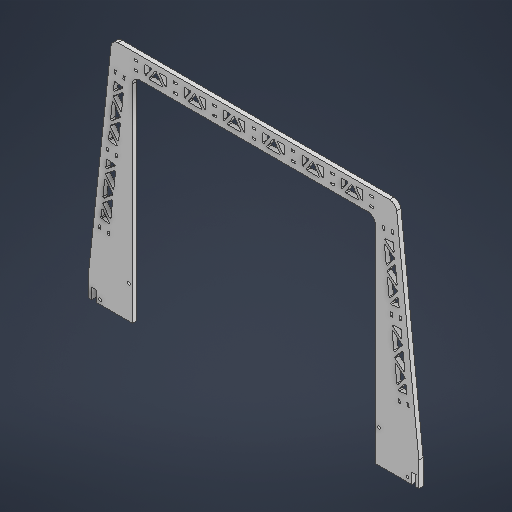
# Autodesk Inventor part: GateBrigeSideLessMaterial
Saved by Autodesk Inventor 2026 (Build 300175000, 175)
## iProperties
Created: 2025-03-30
Part Number: GateBrigeSideLessMaterial
Material: Všeobecné
Document SubType Name: Modeling
Designer: 42060
Density: 1 g/cm^3
Appearance: Výchozí
Author: 42060
Autodesk Inventor part; units mm, degrees
ref_plane "YZ Plane" through (0, 0, 0) normal (1, 0, 0) x (0, 1, 0)
ref_plane "XZ Plane" through (0, 0, 0) normal (0, 1, 0) x (-1, 0, 0)
ref_plane "XY Plane" through (0, 0, 0) normal (0, 0, 1) x (1, 0, 0)
sketch "Náčrt1" plane through (0, 0, 0) normal (0, 0, 1) x (1, 0, 0)
  line L0 (0, 0) -> (-160, 0)
  line L1 (-170, -10) -> (-170, -300)
  line L2 (-231, -300) -> (-231, -265.3)
  line L3 (-190.0581, 30) -> (0, 30)
  line L4 (0, 30) -> (0, 0)
  line L5 (-203.7, -249) -> (-170, -249)
  line L6 (-170, -249) -> (-170, -299)
  line L7 (-170, -299) -> (-220, -299)
  line L8 (-220, -299) -> (-220, -265.3)
  line L9 (-220, -265.3) -> (-203.7, -249)
  line L10 (-220, -299) -> (-170, -249) construction
  circle A0 centre (-215, -294) radius 2.1
  circle A1 centre (-175, -254) radius 2.1
  arc A2 (-160, 0) -> (-170, -10) centre (-160, -10) ccw
  line L11 (-200, 21.0762) -> (-231, -265.3)
  arc A3 (-190.0581, 30) -> (-200, 21.0762) centre (-190.0581, 20) ccw
  line L12 (-227, -300) -> (-227, -285)
  line L13 (-227, -285) -> (-221, -285)
  line L14 (-221, -285) -> (-221, -300)
  line L15 (-170, -300) -> (-221, -300)
  line L16 (-227, -300) -> (-231, -300)
  line L17 (0, 0) -> (160, 0)
  line L18 (170, -10) -> (170, -300)
  line L19 (231, -300) -> (231, -265.3)
  line L20 (190.0581, 30) -> (0, 30)
  line L21 (203.7, -249) -> (170, -249)
  line L22 (170, -249) -> (170, -299)
  line L23 (170, -299) -> (220, -299)
  line L24 (220, -299) -> (220, -265.3)
  line L25 (220, -265.3) -> (203.7, -249)
  line L26 (220, -299) -> (170, -249) construction
  circle A4 centre (215, -294) radius 2.1
  circle A5 centre (175, -254) radius 2.1
  arc A6 (170, -10) -> (160, 0) centre (160, -10) ccw
  line L27 (200, 21.0762) -> (231, -265.3)
  arc A7 (200, 21.0762) -> (190.0581, 30) centre (190.0581, 20) ccw
  line L28 (227, -300) -> (227, -285)
  line L29 (227, -285) -> (221, -285)
  line L30 (221, -285) -> (221, -300)
  line L31 (170, -300) -> (221, -300)
  line L32 (227, -300) -> (231, -300)
  line L33 (-36.6095, 9.0611) -> (-28.3278, 21.2788)
  line L34 (-26.6722, 21.2788) -> (-18.3905, 9.0611)
  line L35 (-19.2183, 7.5) -> (-35.7817, 7.5)
  line L36 (-21.6095, 20.9389) -> (-14.3278, 10.1964)
  line L37 (-12.5, 10.7575) -> (-12.5, 21.5)
  line L38 (-13.5, 22.5) -> (-20.7817, 22.5)
  line L39 (-33.3905, 20.9389) -> (-40.6722, 10.1964)
  line L40 (-42.5, 10.7575) -> (-42.5, 21.5)
  line L41 (-41.5, 22.5) -> (-34.2183, 22.5)
  line L42 (-55, 15) -> (0, 15) construction
  arc A8 (-41.5, 22.5) -> (-42.5, 21.5) centre (-41.5, 21.5) ccw
  arc A9 (-33.3905, 20.9389) -> (-34.2183, 22.5) centre (-34.2183, 21.5) ccw
  arc A10 (-42.5, 10.7575) -> (-40.6722, 10.1964) centre (-41.5, 10.7575) ccw
  arc A11 (-36.6095, 9.0611) -> (-35.7817, 7.5) centre (-35.7817, 8.5) ccw
  arc A12 (-19.2183, 7.5) -> (-18.3905, 9.0611) centre (-19.2183, 8.5) ccw
  arc A13 (-26.6722, 21.2788) -> (-28.3278, 21.2788) centre (-27.5, 20.7178) ccw
  arc A14 (-20.7817, 22.5) -> (-21.6095, 20.9389) centre (-20.7817, 21.5) ccw
  arc A15 (-12.5, 21.5) -> (-13.5, 22.5) centre (-13.5, 21.5) ccw
  arc A16 (-14.3278, 10.1964) -> (-12.5, 10.7575) centre (-13.5, 10.7575) ccw
  arc A17 (-81.6722, 21.2788) -> (-83.3278, 21.2788) centre (-82.5, 20.7178) ccw
  line L43 (-91.6095, 9.0611) -> (-83.3278, 21.2788)
  line L44 (-68.5, 22.5) -> (-75.7817, 22.5)
  arc A18 (-67.5, 21.5) -> (-68.5, 22.5) centre (-68.5, 21.5) ccw
  line L45 (-81.6722, 21.2788) -> (-73.3905, 9.0611)
  arc A19 (-74.2183, 7.5) -> (-73.3905, 9.0611) centre (-74.2183, 8.5) ccw
  line L46 (-76.6095, 20.9389) -> (-69.3278, 10.1964)
  line L47 (-74.2183, 7.5) -> (-90.7817, 7.5)
  arc A20 (-69.3278, 10.1964) -> (-67.5, 10.7575) centre (-68.5, 10.7575) ccw
  line L48 (-110, 15) -> (-55, 15) construction
  arc A21 (-96.5, 22.5) -> (-97.5, 21.5) centre (-96.5, 21.5) ccw
  arc A22 (-97.5, 10.7575) -> (-95.6722, 10.1964) centre (-96.5, 10.7575) ccw
  arc A23 (-91.6095, 9.0611) -> (-90.7817, 7.5) centre (-90.7817, 8.5) ccw
  arc A24 (-88.3905, 20.9389) -> (-89.2183, 22.5) centre (-89.2183, 21.5) ccw
  line L49 (-67.5, 10.7575) -> (-67.5, 21.5)
  arc A25 (-75.7817, 22.5) -> (-76.6095, 20.9389) centre (-75.7817, 21.5) ccw
  line L50 (-96.5, 22.5) -> (-89.2183, 22.5)
  line L51 (-88.3905, 20.9389) -> (-95.6722, 10.1964)
  line L52 (-97.5, 10.7575) -> (-97.5, 21.5)
  arc A26 (-136.6722, 21.2788) -> (-138.3278, 21.2788) centre (-137.5, 20.7178) ccw
  line L53 (-146.6095, 9.0611) -> (-138.3278, 21.2788)
  line L54 (-123.5, 22.5) -> (-130.7817, 22.5)
  arc A27 (-122.5, 21.5) -> (-123.5, 22.5) centre (-123.5, 21.5) ccw
  line L55 (-136.6722, 21.2788) -> (-128.3905, 9.0611)
  arc A28 (-129.2183, 7.5) -> (-128.3905, 9.0611) centre (-129.2183, 8.5) ccw
  line L56 (-131.6095, 20.9389) -> (-124.3278, 10.1964)
  line L57 (-129.2183, 7.5) -> (-145.7817, 7.5)
  arc A29 (-124.3278, 10.1964) -> (-122.5, 10.7575) centre (-123.5, 10.7575) ccw
  line L58 (-165, 15) -> (-110, 15) construction
  arc A30 (-151.5, 22.5) -> (-152.5, 21.5) centre (-151.5, 21.5) ccw
  arc A31 (-152.5, 10.7575) -> (-150.6722, 10.1964) centre (-151.5, 10.7575) ccw
  arc A32 (-146.6095, 9.0611) -> (-145.7817, 7.5) centre (-145.7817, 8.5) ccw
  arc A33 (-143.3905, 20.9389) -> (-144.2183, 22.5) centre (-144.2183, 21.5) ccw
  line L59 (-122.5, 10.7575) -> (-122.5, 21.5)
  arc A34 (-130.7817, 22.5) -> (-131.6095, 20.9389) centre (-130.7817, 21.5) ccw
  line L60 (-151.5, 22.5) -> (-144.2183, 22.5)
  line L61 (-143.3905, 20.9389) -> (-150.6722, 10.1964)
  line L62 (-152.5, 10.7575) -> (-152.5, 21.5)
  line L63 (-194.2882, -19.4076) -> (-184.4169, -20.4762)
  line L64 (-183.8976, -22.2495) -> (-194.8375, -31.0522)
  line L65 (-196.4586, -30.1655) -> (-195.39, -20.2942)
  line L66 (-182.8853, -28.7602) -> (-185.2377, -50.4911)
  line L67 (-187.011, -51.0104) -> (-196.7003, -38.9688)
  line L68 (-196.5481, -37.5628) -> (-184.5064, -27.8735)
  line L69 (-196.4225, -45.6946) -> (-186.7332, -57.7362)
  line L70 (-186.8854, -59.1422) -> (-198.927, -68.8315)
  line L71 (-200.5481, -67.9448) -> (-198.1958, -46.2139)
  line L72 (-188.596, -65.6528) -> (-200.6376, -75.3421)
  line L73 (-200.7898, -76.7481) -> (-191.1006, -88.7897)
  line L74 (-189.3273, -88.2704) -> (-186.9749, -66.5395)
  line L75 (-200.5121, -83.4739) -> (-191.7094, -94.4137)
  line L76 (-192.5961, -96.0348) -> (-202.4673, -94.9662)
  line L77 (-203.3539, -93.8644) -> (-202.2854, -83.9932)
  line L78 (-189.3526, -19.9419) -> (-188.3302, -10.4971) construction
  arc A35 (-194.2882, -19.4076) -> (-195.39, -20.2942) centre (-194.3958, -20.4018) ccw
  arc A36 (-183.8976, -22.2495) -> (-184.4169, -20.4762) centre (-184.5245, -21.4704) ccw
  arc A37 (-196.4586, -30.1655) -> (-194.8375, -31.0522) centre (-195.4644, -30.2731) ccw
  arc A38 (-196.5481, -37.5628) -> (-196.7003, -38.9688) centre (-195.9212, -38.3419) ccw
  arc A39 (-187.011, -51.0104) -> (-185.2377, -50.4911) centre (-186.2319, -50.3835) ccw
  arc A40 (-182.8853, -28.7602) -> (-184.5064, -27.8735) centre (-183.8795, -28.6526) ccw
  arc A41 (-196.4225, -45.6946) -> (-198.1958, -46.2139) centre (-197.2016, -46.3215) ccw
  arc A42 (-186.8854, -59.1422) -> (-186.7332, -57.7362) centre (-187.5123, -58.3631) ccw
  arc A43 (-200.5481, -67.9448) -> (-198.927, -68.8315) centre (-199.5539, -68.0524) ccw
  arc A44 (-200.6376, -75.3421) -> (-200.7898, -76.7481) centre (-200.0107, -76.1212) ccw
  arc A45 (-191.1006, -88.7897) -> (-189.3273, -88.2704) centre (-190.3215, -88.1628) ccw
  arc A46 (-186.9749, -66.5395) -> (-188.596, -65.6528) centre (-187.9691, -66.4319) ccw
  arc A47 (-200.5121, -83.4739) -> (-202.2854, -83.9932) centre (-201.2912, -84.1008) ccw
  arc A48 (-203.3539, -93.8644) -> (-202.4673, -94.9662) centre (-202.3597, -93.972) ccw
  arc A49 (-192.5961, -96.0348) -> (-191.7094, -94.4137) centre (-192.4885, -95.0406) ccw
  arc A50 (-214.116, -193.2836) -> (-213.2294, -194.3854) centre (-213.1218, -193.3913) ccw
  line L79 (-203.3581, -195.454) -> (-213.2294, -194.3854)
  arc A51 (-203.3581, -195.454) -> (-202.4714, -193.8329) centre (-203.2505, -194.4598) ccw
  arc A52 (-201.8626, -188.2089) -> (-200.0893, -187.6896) centre (-201.0835, -187.582) ccw
  line L80 (-211.2741, -182.8931) -> (-202.4714, -193.8329)
  line L81 (-214.116, -193.2836) -> (-213.0474, -183.4124)
  arc A53 (-211.2741, -182.8931) -> (-213.0474, -183.4124) centre (-212.0532, -183.52) ccw
  line L82 (-199.3581, -165.072) -> (-211.3997, -174.7613)
  line L83 (-211.5519, -176.1673) -> (-201.8626, -188.2089)
  line L84 (-200.0893, -187.6896) -> (-197.737, -165.9587)
  arc A54 (-211.3997, -174.7613) -> (-211.5519, -176.1673) centre (-210.7728, -175.5404) ccw
  arc A55 (-211.3102, -167.364) -> (-209.6891, -168.2507) centre (-210.316, -167.4716) ccw
  arc A56 (-197.737, -165.9587) -> (-199.3581, -165.072) centre (-198.7312, -165.8511) ccw
  line L85 (-207.1845, -145.1138) -> (-197.4953, -157.1554)
  arc A57 (-197.6475, -158.5614) -> (-197.4953, -157.1554) centre (-198.2744, -157.7823) ccw
  line L86 (-211.3102, -167.364) -> (-208.9578, -145.6331)
  line L87 (-197.6475, -158.5614) -> (-209.6891, -168.2507)
  arc A58 (-197.773, -150.4296) -> (-195.9997, -149.9103) centre (-196.9939, -149.8027) ccw
  arc A59 (-207.1845, -145.1138) -> (-208.9578, -145.6331) centre (-207.9636, -145.7407) ccw
  line L88 (-197.773, -150.4296) -> (-207.4623, -138.388)
  arc A60 (-207.3101, -136.982) -> (-207.4623, -138.388) centre (-206.6832, -137.7611) ccw
  arc A61 (-207.2206, -129.5847) -> (-205.5995, -130.4714) centre (-206.2264, -129.6923) ccw
  line L89 (-193.6474, -128.1794) -> (-195.9997, -149.9103)
  line L90 (-207.3101, -136.982) -> (-195.2685, -127.2927)
  arc A62 (-193.6474, -128.1794) -> (-195.2685, -127.2927) centre (-194.6416, -128.0718) ccw
  arc A63 (-194.6597, -121.6687) -> (-195.179, -119.8954) centre (-195.2866, -120.8896) ccw
  line L91 (-200.1146, -119.3611) -> (-199.0922, -109.9163) construction
  line L92 (-205.0502, -118.8268) -> (-195.179, -119.8954)
  arc A64 (-205.0502, -118.8268) -> (-206.152, -119.7134) centre (-205.1579, -119.821) ccw
  line L93 (-194.6597, -121.6687) -> (-205.5995, -130.4714)
  line L94 (-207.2206, -129.5847) -> (-206.152, -119.7134)
  line L95 (36.6095, 9.0611) -> (28.3278, 21.2788)
  line L96 (26.6722, 21.2788) -> (18.3905, 9.0611)
  line L97 (19.2183, 7.5) -> (35.7817, 7.5)
  line L98 (21.6095, 20.9389) -> (14.3278, 10.1964)
  line L99 (12.5, 10.7575) -> (12.5, 21.5)
  line L100 (13.5, 22.5) -> (20.7817, 22.5)
  line L101 (33.3905, 20.9389) -> (40.6722, 10.1964)
  line L102 (42.5, 10.7575) -> (42.5, 21.5)
  line L103 (41.5, 22.5) -> (34.2183, 22.5)
  line L104 (55, 15) -> (0, 15) construction
  arc A65 (42.5, 21.5) -> (41.5, 22.5) centre (41.5, 21.5) ccw
  arc A66 (34.2183, 22.5) -> (33.3905, 20.9389) centre (34.2183, 21.5) ccw
  arc A67 (40.6722, 10.1964) -> (42.5, 10.7575) centre (41.5, 10.7575) ccw
  arc A68 (35.7817, 7.5) -> (36.6095, 9.0611) centre (35.7817, 8.5) ccw
  arc A69 (18.3905, 9.0611) -> (19.2183, 7.5) centre (19.2183, 8.5) ccw
  arc A70 (28.3278, 21.2788) -> (26.6722, 21.2788) centre (27.5, 20.7178) ccw
  arc A71 (21.6095, 20.9389) -> (20.7817, 22.5) centre (20.7817, 21.5) ccw
  arc A72 (13.5, 22.5) -> (12.5, 21.5) centre (13.5, 21.5) ccw
  arc A73 (12.5, 10.7575) -> (14.3278, 10.1964) centre (13.5, 10.7575) ccw
  line L105 (67.5, 10.7575) -> (67.5, 21.5)
  line L106 (96.5, 22.5) -> (89.2183, 22.5)
  arc A74 (97.5, 21.5) -> (96.5, 22.5) centre (96.5, 21.5) ccw
  line L107 (97.5, 10.7575) -> (97.5, 21.5)
  arc A75 (95.6722, 10.1964) -> (97.5, 10.7575) centre (96.5, 10.7575) ccw
  arc A76 (67.5, 10.7575) -> (69.3278, 10.1964) centre (68.5, 10.7575) ccw
  arc A77 (68.5, 22.5) -> (67.5, 21.5) centre (68.5, 21.5) ccw
  arc A78 (89.2183, 22.5) -> (88.3905, 20.9389) centre (89.2183, 21.5) ccw
  arc A79 (83.3278, 21.2788) -> (81.6722, 21.2788) centre (82.5, 20.7178) ccw
  line L108 (88.3905, 20.9389) -> (95.6722, 10.1964)
  line L109 (91.6095, 9.0611) -> (83.3278, 21.2788)
  arc A80 (76.6095, 20.9389) -> (75.7817, 22.5) centre (75.7817, 21.5) ccw
  arc A81 (90.7817, 7.5) -> (91.6095, 9.0611) centre (90.7817, 8.5) ccw
  line L110 (110, 15) -> (55, 15) construction
  line L111 (68.5, 22.5) -> (75.7817, 22.5)
  line L112 (76.6095, 20.9389) -> (69.3278, 10.1964)
  line L113 (81.6722, 21.2788) -> (73.3905, 9.0611)
  arc A82 (73.3905, 9.0611) -> (74.2183, 7.5) centre (74.2183, 8.5) ccw
  line L114 (74.2183, 7.5) -> (90.7817, 7.5)
  line L115 (122.5, 10.7575) -> (122.5, 21.5)
  line L116 (151.5, 22.5) -> (144.2183, 22.5)
  arc A83 (152.5, 21.5) -> (151.5, 22.5) centre (151.5, 21.5) ccw
  line L117 (152.5, 10.7575) -> (152.5, 21.5)
  arc A84 (150.6722, 10.1964) -> (152.5, 10.7575) centre (151.5, 10.7575) ccw
  arc A85 (122.5, 10.7575) -> (124.3278, 10.1964) centre (123.5, 10.7575) ccw
  arc A86 (123.5, 22.5) -> (122.5, 21.5) centre (123.5, 21.5) ccw
  arc A87 (144.2183, 22.5) -> (143.3905, 20.9389) centre (144.2183, 21.5) ccw
  arc A88 (138.3278, 21.2788) -> (136.6722, 21.2788) centre (137.5, 20.7178) ccw
  line L118 (143.3905, 20.9389) -> (150.6722, 10.1964)
  line L119 (146.6095, 9.0611) -> (138.3278, 21.2788)
  arc A89 (131.6095, 20.9389) -> (130.7817, 22.5) centre (130.7817, 21.5) ccw
  arc A90 (145.7817, 7.5) -> (146.6095, 9.0611) centre (145.7817, 8.5) ccw
  line L120 (165, 15) -> (110, 15) construction
  line L121 (123.5, 22.5) -> (130.7817, 22.5)
  line L122 (131.6095, 20.9389) -> (124.3278, 10.1964)
  line L123 (136.6722, 21.2788) -> (128.3905, 9.0611)
  arc A91 (128.3905, 9.0611) -> (129.2183, 7.5) centre (129.2183, 8.5) ccw
  line L124 (129.2183, 7.5) -> (145.7817, 7.5)
  line L125 (194.2882, -19.4076) -> (184.4169, -20.4762)
  line L126 (183.8976, -22.2495) -> (194.8375, -31.0522)
  line L127 (196.4586, -30.1655) -> (195.39, -20.2942)
  line L128 (182.8853, -28.7602) -> (185.2377, -50.4911)
  line L129 (187.011, -51.0104) -> (196.7003, -38.9688)
  line L130 (196.5481, -37.5628) -> (184.5064, -27.8735)
  line L131 (196.4225, -45.6946) -> (186.7332, -57.7362)
  line L132 (186.8854, -59.1422) -> (198.927, -68.8315)
  line L133 (200.5481, -67.9448) -> (198.1958, -46.2139)
  line L134 (188.596, -65.6528) -> (200.6376, -75.3421)
  line L135 (200.7898, -76.7481) -> (191.1006, -88.7897)
  line L136 (189.3273, -88.2704) -> (186.9749, -66.5395)
  line L137 (200.5121, -83.4739) -> (191.7094, -94.4137)
  line L138 (192.5961, -96.0348) -> (202.4673, -94.9662)
  line L139 (203.3539, -93.8644) -> (202.2854, -83.9932)
  arc A92 (195.39, -20.2942) -> (194.2882, -19.4076) centre (194.3958, -20.4018) ccw
  arc A93 (184.4169, -20.4762) -> (183.8976, -22.2495) centre (184.5245, -21.4704) ccw
  arc A94 (194.8375, -31.0522) -> (196.4586, -30.1655) centre (195.4644, -30.2731) ccw
  arc A95 (196.7003, -38.9688) -> (196.5481, -37.5628) centre (195.9212, -38.3419) ccw
  arc A96 (185.2377, -50.4911) -> (187.011, -51.0104) centre (186.2319, -50.3835) ccw
  arc A97 (184.5064, -27.8735) -> (182.8853, -28.7602) centre (183.8795, -28.6526) ccw
  arc A98 (198.1958, -46.2139) -> (196.4225, -45.6946) centre (197.2016, -46.3215) ccw
  arc A99 (186.7332, -57.7362) -> (186.8854, -59.1422) centre (187.5123, -58.3631) ccw
  arc A100 (198.927, -68.8315) -> (200.5481, -67.9448) centre (199.5539, -68.0524) ccw
  arc A101 (200.7898, -76.7481) -> (200.6376, -75.3421) centre (200.0107, -76.1212) ccw
  arc A102 (189.3273, -88.2704) -> (191.1006, -88.7897) centre (190.3215, -88.1628) ccw
  arc A103 (188.596, -65.6528) -> (186.9749, -66.5395) centre (187.9691, -66.4319) ccw
  arc A104 (202.2854, -83.9932) -> (200.5121, -83.4739) centre (201.2912, -84.1008) ccw
  arc A105 (202.4673, -94.9662) -> (203.3539, -93.8644) centre (202.3597, -93.972) ccw
  arc A106 (191.7094, -94.4137) -> (192.5961, -96.0348) centre (192.4885, -95.0406) ccw
  arc A107 (195.179, -119.8954) -> (194.6597, -121.6687) centre (195.2866, -120.8896) ccw
  arc A108 (195.2685, -127.2927) -> (193.6474, -128.1794) centre (194.6416, -128.0718) ccw
  line L140 (205.0502, -118.8268) -> (195.179, -119.8954)
  line L141 (194.6597, -121.6687) -> (205.5995, -130.4714)
  line L142 (207.2206, -129.5847) -> (206.152, -119.7134)
  line L143 (207.3101, -136.982) -> (195.2685, -127.2927)
  arc A109 (206.152, -119.7134) -> (205.0502, -118.8268) centre (205.1579, -119.821) ccw
  arc A110 (205.5995, -130.4714) -> (207.2206, -129.5847) centre (206.2264, -129.6923) ccw
  line L144 (193.6474, -128.1794) -> (195.9997, -149.9103)
  arc A111 (208.9578, -145.6331) -> (207.1845, -145.1138) centre (207.9636, -145.7407) ccw
  line L145 (197.773, -150.4296) -> (207.4623, -138.388)
  arc A112 (207.4623, -138.388) -> (207.3101, -136.982) centre (206.6832, -137.7611) ccw
  arc A113 (195.9997, -149.9103) -> (197.773, -150.4296) centre (196.9939, -149.8027) ccw
  line L146 (207.1845, -145.1138) -> (197.4953, -157.1554)
  arc A114 (197.4953, -157.1554) -> (197.6475, -158.5614) centre (198.2744, -157.7823) ccw
  arc A115 (199.3581, -165.072) -> (197.737, -165.9587) centre (198.7312, -165.8511) ccw
  line L147 (197.6475, -158.5614) -> (209.6891, -168.2507)
  arc A116 (209.6891, -168.2507) -> (211.3102, -167.364) centre (210.316, -167.4716) ccw
  line L148 (211.3102, -167.364) -> (208.9578, -145.6331)
  arc A117 (202.4714, -193.8329) -> (203.3581, -195.454) centre (203.2505, -194.4598) ccw
  arc A118 (213.2294, -194.3854) -> (214.116, -193.2836) centre (213.1218, -193.3913) ccw
  arc A119 (200.0893, -187.6896) -> (201.8626, -188.2089) centre (201.0835, -187.582) ccw
  line L149 (214.116, -193.2836) -> (213.0474, -183.4124)
  line L150 (211.2741, -182.8931) -> (202.4714, -193.8329)
  arc A120 (213.0474, -183.4124) -> (211.2741, -182.8931) centre (212.0532, -183.52) ccw
  line L151 (211.5519, -176.1673) -> (201.8626, -188.2089)
  arc A121 (211.5519, -176.1673) -> (211.3997, -174.7613) centre (210.7728, -175.5404) ccw
  line L152 (200.0893, -187.6896) -> (197.737, -165.9587)
  line L153 (199.3581, -165.072) -> (211.3997, -174.7613)
  line L154 (203.3581, -195.454) -> (213.2294, -194.3854)
  line L155 (-2.5, 10) -> (2.5, 10)
  line L156 (2.5, 10) -> (2.5, 7.5)
  line L157 (2.5, 7.5) -> (-2.5, 7.5)
  line L158 (-2.5, 7.5) -> (-2.5, 10)
  line L159 (-2.5, 22.5) -> (2.5, 22.5)
  line L160 (2.5, 22.5) -> (2.5, 20)
  line L161 (2.5, 20) -> (-2.5, 20)
  line L162 (-2.5, 20) -> (-2.5, 22.5)
  line L163 (0, 20) -> (0, 10) construction
  line L164 (-42.5, 10.7575) -> (-42.5, 7.5) construction
  line L165 (-42.5, 7.5) -> (-40.6722, 10.1964) construction
  line L166 (-27.5, 22.5) -> (-27.5, 7.5) construction
  line L167 (-52.5, 10) -> (-52.5, 7.5)
  line L168 (-57.5, 10) -> (-52.5, 10)
  line L169 (-52.5, 7.5) -> (-57.5, 7.5)
  line L170 (-57.5, 7.5) -> (-57.5, 10)
  line L171 (-57.5, 22.5) -> (-52.5, 22.5)
  line L172 (-52.5, 20) -> (-57.5, 20)
  line L173 (-57.5, 20) -> (-57.5, 22.5)
  line L174 (-52.5, 22.5) -> (-52.5, 20)
  line L175 (-107.5, 10) -> (-107.5, 7.5)
  line L176 (-112.5, 10) -> (-107.5, 10)
  line L177 (-107.5, 7.5) -> (-112.5, 7.5)
  line L178 (-112.5, 7.5) -> (-112.5, 10)
  line L179 (-112.5, 22.5) -> (-107.5, 22.5)
  line L180 (-107.5, 20) -> (-112.5, 20)
  line L181 (-112.5, 20) -> (-112.5, 22.5)
  line L182 (-107.5, 22.5) -> (-107.5, 20)
  line L183 (-162.5, 10) -> (-162.5, 7.5)
  line L184 (-167.5, 10) -> (-162.5, 10)
  line L185 (-162.5, 7.5) -> (-167.5, 7.5)
  line L186 (-167.5, 7.5) -> (-167.5, 10)
  line L187 (-167.5, 22.5) -> (-162.5, 22.5)
  line L188 (-162.5, 20) -> (-167.5, 20)
  line L189 (-167.5, 20) -> (-167.5, 22.5)
  line L190 (-162.5, 22.5) -> (-162.5, 20)
  line L191 (52.5, 20) -> (52.5, 22.5)
  line L192 (57.5, 20) -> (52.5, 20)
  line L193 (57.5, 22.5) -> (57.5, 20)
  line L194 (52.5, 22.5) -> (57.5, 22.5)
  line L195 (57.5, 10) -> (57.5, 7.5)
  line L196 (52.5, 10) -> (57.5, 10)
  line L197 (57.5, 7.5) -> (52.5, 7.5)
  line L198 (52.5, 7.5) -> (52.5, 10)
  line L199 (107.5, 20) -> (107.5, 22.5)
  line L200 (112.5, 20) -> (107.5, 20)
  line L201 (112.5, 22.5) -> (112.5, 20)
  line L202 (107.5, 22.5) -> (112.5, 22.5)
  line L203 (112.5, 10) -> (112.5, 7.5)
  line L204 (107.5, 10) -> (112.5, 10)
  line L205 (112.5, 7.5) -> (107.5, 7.5)
  line L206 (107.5, 7.5) -> (107.5, 10)
  line L207 (162.5, 20) -> (162.5, 22.5)
  line L208 (167.5, 20) -> (162.5, 20)
  line L209 (167.5, 22.5) -> (167.5, 20)
  line L210 (162.5, 22.5) -> (167.5, 22.5)
  line L211 (167.5, 10) -> (167.5, 7.5)
  line L212 (162.5, 10) -> (167.5, 10)
  line L213 (167.5, 7.5) -> (162.5, 7.5)
  line L214 (162.5, 7.5) -> (162.5, 10)
  line L215 (-195.2485, -4.719) -> (-192.763, -4.988)
  line L216 (-192.763, -4.988) -> (-193.3011, -9.959)
  line L217 (-193.3011, -9.959) -> (-195.7866, -9.6899)
  line L218 (-195.7866, -9.6899) -> (-195.2485, -4.719)
  line L219 (-182.8211, -6.0642) -> (-180.3356, -6.3333)
  line L220 (-180.3356, -6.3333) -> (-180.8737, -11.3042)
  line L221 (-180.8737, -11.3042) -> (-183.3592, -11.0352)
  line L222 (-183.3592, -11.0352) -> (-182.8211, -6.0642)
  line L223 (-193.3011, -9.959) -> (-183.3592, -11.0352) construction
  line L224 (-206.5486, -109.1091) -> (-206.0105, -104.1382)
  line L225 (-203.5251, -104.4072) -> (-204.0632, -109.3782)
  line L226 (-204.0632, -109.3782) -> (-206.5486, -109.1091)
  line L227 (-206.0105, -104.1382) -> (-203.5251, -104.4072)
  line L228 (-194.1212, -110.4544) -> (-193.5831, -105.4834)
  line L229 (-191.6358, -110.7235) -> (-194.1212, -110.4544)
  line L230 (-191.0977, -105.7525) -> (-191.6358, -110.7235)
  line L231 (-193.5831, -105.4834) -> (-191.0977, -105.7525)
  line L232 (-204.0632, -109.3782) -> (-194.1212, -110.4544) construction
  line L233 (-203.5251, -104.4072) -> (-193.5831, -105.4834) construction
  line L234 (-198.6079, -105.4424) -> (-197.5317, -95.5005) construction
  line L235 (-217.3107, -208.5284) -> (-216.7726, -203.5574)
  line L236 (-214.2871, -203.8264) -> (-214.8252, -208.7974)
  line L237 (-214.8252, -208.7974) -> (-217.3107, -208.5284)
  line L238 (-216.7726, -203.5574) -> (-214.2871, -203.8264)
  line L239 (-204.8833, -209.8736) -> (-204.3452, -204.9026)
  line L240 (-202.3978, -210.1427) -> (-204.8833, -209.8736)
  line L241 (-201.8597, -205.1717) -> (-202.3978, -210.1427)
  line L242 (-204.3452, -204.9026) -> (-201.8597, -205.1717)
  line L243 (-214.8252, -208.7974) -> (-204.8833, -209.8736) construction
  line L244 (195.2485, -4.719) -> (192.763, -4.988)
  line L245 (192.763, -4.988) -> (193.3011, -9.959)
  line L246 (193.3011, -9.959) -> (195.7866, -9.6899)
  line L247 (195.7866, -9.6899) -> (195.2485, -4.719)
  line L248 (182.8211, -6.0642) -> (180.3356, -6.3333)
  line L249 (180.3356, -6.3333) -> (180.8737, -11.3042)
  line L250 (180.8737, -11.3042) -> (183.3592, -11.0352)
  line L251 (183.3592, -11.0352) -> (182.8211, -6.0642)
  line L252 (206.5486, -109.1091) -> (206.0105, -104.1382)
  line L253 (203.5251, -104.4072) -> (204.0632, -109.3782)
  line L254 (204.0632, -109.3782) -> (206.5486, -109.1091)
  line L255 (206.0105, -104.1382) -> (203.5251, -104.4072)
  line L256 (194.1212, -110.4544) -> (193.5831, -105.4834)
  line L257 (191.6358, -110.7235) -> (194.1212, -110.4544)
  line L258 (191.0977, -105.7525) -> (191.6358, -110.7235)
  line L259 (193.5831, -105.4834) -> (191.0977, -105.7525)
  line L260 (217.3107, -208.5284) -> (216.7726, -203.5574)
  line L261 (214.2871, -203.8264) -> (214.8252, -208.7974)
  line L262 (214.8252, -208.7974) -> (217.3107, -208.5284)
  line L263 (216.7726, -203.5574) -> (214.2871, -203.8264)
  line L264 (204.8833, -209.8736) -> (204.3452, -204.9026)
  line L265 (202.3978, -210.1427) -> (204.8833, -209.8736)
  line L266 (201.8597, -205.1717) -> (202.3978, -210.1427)
  line L267 (204.3452, -204.9026) -> (201.8597, -205.1717)
  line L268 (-188.3302, -10.4971) -> (-188.2763, -10) construction
  point P0 (-12.5, 7.5)
  point P1 (-32.3323, 22.5)
  point P2 (-42.5, 22.5)
  point P3 (-27.5, 15)
  point P4 (-12.5, 16.1288)
  point P5 (-82.5, 22.5)
  point P6 (-82.5, 15)
  point P7 (-82.5, 7.5)
  point P8 (-87.3323, 22.5)
  point P9 (-97.5, 22.5)
  point P10 (-67.5, 7.5)
  point P11 (-67.5, 16.1288)
  point P12 (-137.5, 22.5)
  point P13 (-137.5, 15)
  point P14 (-137.5, 7.5)
  point P15 (-142.3323, 22.5)
  point P16 (-152.5, 22.5)
  point P17 (-122.5, 7.5)
  point P18 (-122.5, 16.1288)
  point P19 (-195.2824, -19.3)
  point P20 (-182.0167, -20.736)
  point P21 (-196.7184, -32.5657)
  point P22 (-182.6255, -26.36)
  point P23 (-185.4975, -52.8913)
  point P24 (-197.3272, -38.1897)
  point P25 (-197.936, -43.8137)
  point P26 (-186.1063, -58.5153)
  point P27 (-200.808, -70.345)
  point P28 (-186.7151, -64.1393)
  point P29 (-201.4167, -75.969)
  point P30 (-189.5871, -90.6706)
  point P31 (-202.0255, -81.593)
  point P32 (-190.1959, -96.2946)
  point P33 (-203.4615, -94.8586)
  point P34 (-214.2236, -194.2778)
  point P35 (-200.9579, -195.7138)
  point P36 (-200.3491, -190.0898)
  point P37 (-212.7876, -181.0122)
  point P38 (-212.1788, -175.3882)
  point P39 (-211.57, -169.7642)
  point P40 (-197.4772, -163.5585)
  point P41 (-196.8684, -157.9345)
  point P42 (-196.2596, -152.3105)
  point P43 (-208.698, -143.2329)
  point P44 (-208.0892, -137.6089)
  point P45 (-207.4804, -131.9849)
  point P46 (-193.3876, -125.7792)
  point P47 (-192.7788, -120.1552)
  point P48 (-206.0444, -118.7192)
  point P49 (27.5, 22.5)
  point P50 (12.5, 7.5)
  point P51 (32.3323, 22.5)
  point P52 (42.5, 22.5)
  point P53 (27.5, 7.5)
  point P54 (27.5, 15)
  point P55 (12.5, 16.1288)
  point P56 (67.5, 7.5)
  point P57 (67.5, 16.1288)
  point P58 (82.5, 22.5)
  point P59 (87.3323, 22.5)
  point P60 (97.5, 22.5)
  point P61 (82.5, 15)
  point P62 (82.5, 7.5)
  point P63 (122.5, 7.5)
  point P64 (122.5, 16.1288)
  point P65 (137.5, 22.5)
  point P66 (142.3323, 22.5)
  point P67 (152.5, 22.5)
  point P68 (137.5, 15)
  point P69 (137.5, 7.5)
  point P70 (195.2824, -19.3)
  point P71 (182.0167, -20.736)
  point P72 (196.7184, -32.5657)
  point P73 (182.6255, -26.36)
  point P74 (185.4975, -52.8913)
  point P75 (197.3272, -38.1897)
  point P76 (197.936, -43.8137)
  point P77 (186.1063, -58.5153)
  point P78 (200.808, -70.345)
  point P79 (186.7151, -64.1393)
  point P80 (201.4167, -75.969)
  point P81 (189.5871, -90.6706)
  point P82 (202.0255, -81.593)
  point P83 (190.1959, -96.2946)
  point P84 (203.4615, -94.8586)
  point P85 (189.3526, -19.9419)
  point P86 (192.7788, -120.1552)
  point P87 (193.3876, -125.7792)
  point P88 (200.1146, -119.3611)
  point P89 (206.0444, -118.7192)
  point P90 (207.4804, -131.9849)
  point P91 (208.0892, -137.6089)
  point P92 (196.2596, -152.3105)
  point P93 (208.698, -143.2329)
  point P94 (196.8684, -157.9345)
  point P95 (197.4772, -163.5585)
  point P96 (211.57, -169.7642)
  point P97 (214.2236, -194.2778)
  point P98 (200.9579, -195.7138)
  point P99 (200.3491, -190.0898)
  point P100 (212.1788, -175.3882)
  point P101 (212.7876, -181.0122)
  point P102 (0, 15)
  point P103 (-27.5, 15)
  point P104 (-55, 10)
  point P105 (-55, 20)
  point P106 (-110, 10)
  point P107 (-110, 20)
  point P108 (-165, 10)
  point P109 (-165, 20)
  point P110 (55, 20)
  point P111 (55, 10)
  point P112 (110, 20)
  point P113 (110, 10)
  point P114 (165, 20)
  point P115 (165, 10)
  point P116 (-209.8543, -209.3355)
  point P117 (-198.5541, -104.9453)
  dimension "d0" = 50
  dimension "d1" = 50
  dimension "d3" = 33.7
  dimension "d4" = 45
  dimension "d5" = 0
  dimension "d6" = 4.2
  dimension "d7" = 5
  dimension "d8" = 5
  dimension "d10" = 170
  dimension "d12" = 30
  dimension "d14" = 10
  dimension "d16" = 15
  dimension "d17" = 1
  dimension "d18" = 6
  dimension "d19" = 1
  dimension "d20" = 4
  dimension "d21" = 300
  dimension "d22" = 30
  dimension "d46" = 4
  dimension "d47" = 4
  dimension "d50" = 15
  dimension "d51" = 30
  dimension "d52" = 1
  dimension "d55" = 55
  dimension "d63" = 4
  dimension "d64" = 4
  dimension "d65" = 4
  dimension "d66" = 4
  dimension "d67" = 1
  dimension "d70" = 100
  dimension "d77" = 55
  dimension "d84" = 100
  dimension "d91" = 2.5
  dimension "d92" = 5
  dimension "d93" = 15
  dimension "d96" = 55
  dimension "d103" = 55
  dimension "d108" = 5
  dimension "d109" = 2.5
  dimension "d110" = 7.5
  dimension "d111" = 15
  dimension "d115" = 100
  dimension "d123" = 0.5
  dimension "d124" = 0.5
  dimension "d125" = 10
  dimension "d126" = 10
  constraints: 538 end point, 236 point on circle, 227 point on line, 141 symmetric about line, 122 centre point, 52 tangent, 24 equal radius, 24 perpendicular, 20 parallel, 12 midpoint, 11 collinear, 10 coincident, 10 horizontal, 5 equal length, 4 horizontal alignment, 4 vertical alignment, 2 vertical, 579 other
  measures "d0" distance of L5.end L6.end
  measures "d1" distance of L6.end L7.end
  measures "d3" distance of L5.start L5.end
  measures "d4" angle of L5 L9
  measures "d5" distance between parallel lines of L1 L6
  measures "d6" diameter of A1
  measures "d7" distance from line of L5 A1.centre
  measures "d8" distance from line of L7 A0.centre
  measures "d10" distance between parallel lines of L1 L4
  measures "d12" distance between parallel lines of L0 L3
  measures "d14" radius of A3
  measures "d16" distance between parallel lines of L16 L13
  measures "d17" distance between parallel lines of L7 L15
  measures "d18" distance between parallel lines of L14 L12
  measures "d19" distance between parallel lines of L8 L14
  measures "d20" distance between parallel lines of L12 L2
  measures "d21" distance between parallel lines of L15 L0
  measures "d22" distance from line of L11.start L1
  measures "d46" distance between parallel lines of L33 L39
  measures "d47" distance between parallel lines of L36 L34
  measures "d50" distance from line of L35 L166.start
  measures "d51" distance between parallel lines of L37 L40
  measures "d52" radius of A8
  measures "d55" distance of L166.start point (-82.5, 22.5)
  measures "d63" distance between parallel lines of L68 L64
  measures "d64" distance between parallel lines of L69 L67
  measures "d65" distance between parallel lines of L72 L70
  measures "d66" distance between parallel lines of L73 L75
  measures "d67" radius of A35
  measures "d70" distance of point (-203.462, -94.859) point (-214.224, -194.278)
  measures "d77" distance of point (12.5, 7.5) point (67.5, 7.5)
  measures "d84" distance of point (182.017, -20.736) point (192.779, -120.155)
  measures "d91" distance of L159.end L160.end
  measures "d92" distance of L159.start L159.end
  measures "d93" distance between parallel lines of L157 L159
  measures "d96" distance of L155.end L167.start
  measures "d103" distance of L159.start L191.end
  measures "d108" distance of L217.end L215.start
  measures "d109" distance of L215.start L215.end
  measures "d110" distance between parallel lines of L11 L218
  measures "d111" distance between parallel lines of L220 L218
  measures "d115" distance of L217.end L224.start
  measures "d123" distance of L268.start L268.end
  measures "d124" distance from line of L234.start L233
  measures "d125" distance of L78.start L268.end
  measures "d126" distance of L234.start L234.end
extrude "Vysunutí1" add sketch "Náčrt1" along normal blind 6 contours L0 A2 L1 L5 L9 L8 L7 L15 L14 L13 L12 L16 L2 L11 A3 L3 L4 L159 L162 L161 L155 L158 L157 | L4 L157 L156 L155 L161 L160 L159 L20 A7 L27 L19 L32 L28 L29 L30 L31 L18 L23 L24 L25 L21 A6 L17 | L1 L7 L8 L9 L5 | L21 L25 L24 L23 L18
equation "\"d44\" = d18"
